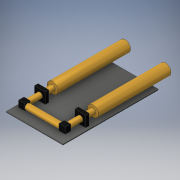
# Autodesk Inventor part: Cannon Barrel
Saved by Autodesk Inventor 2016 (Build 200138000, 138)
## iProperties
Created: 2018-05-17
Part Number: Cannon Barrel
Material: Generic
Document SubType Name: Modeling
Designer: Kade
Density: 1 g/cm^3
Appearance: Default
Mass: 6981.81 g
Surface Area: 8261.67 cm^2
Volume: 6981.81 cm^3
Author: Kade
Autodesk Inventor part; units mm, degrees
ref_plane "YZ Plane" through (0, 0, 0) normal (1, 0, 0) x (0, 1, 0)
ref_plane "XZ Plane" through (0, 0, 0) normal (0, 1, 0) x (-1, 0, 0)
ref_plane "XY Plane" through (0, 0, 0) normal (0, 0, 1) x (1, 0, 0)
sketch "Sketch1" plane through (0, 0, 0) normal (0, 1, 0) x (-1, 0, 0)
  line L0 (198.4375, 333.375) -> (198.4375, -333.375)
  line L1 (198.4375, -333.375) -> (-198.4375, -333.375)
  line L2 (-198.4375, -333.375) -> (-198.4375, 333.375)
  line L3 (-198.4375, 333.375) -> (198.4375, 333.375)
  line L4 (198.4375, 333.375) -> (-198.4375, -333.375) construction
  line L5 (198.4375, -333.375) -> (-198.4375, 333.375) construction
  point P0 (0, 0)
  dimension "d0" = 666.75
  dimension "d1" = 396.875
  constraints: 12 end point, 2 midpoint, 2 parallel, 1 perpendicular, 1 vertical
  measures "d0" distance of L0.start L0.end
  measures "d1" distance of L0.end L1.end
extrude "Extrusion1" add sketch "Sketch1" along normal blind 6.35
sketch "Sketch2" plane through (0, 6.35, 0) normal (0, 1, 0) x (1, 0, 0)
  line L0 (179.3875, -155.575) -> (103.1875, -155.575)
  line L1 (103.1875, -155.575) -> (103.1875, -130.175)
  line L2 (103.1875, -130.175) -> (179.3875, -130.175)
  line L3 (179.3875, -130.175) -> (179.3875, -155.575)
  line L4 (198.4375, -333.375) -> (198.4375, 333.375) projected
  line L5 (-179.3875, -155.575) -> (-103.1875, -155.575)
  line L6 (-103.1875, -155.575) -> (-103.1875, -130.175)
  line L7 (-103.1875, -130.175) -> (-179.3875, -130.175)
  line L8 (-179.3875, -130.175) -> (-179.3875, -155.575)
  line L9 (-198.4375, 333.375) -> (-198.4375, -333.375) projected
  line L10 (198.4375, -333.375) -> (-198.4375, -333.375) projected
  point P0 (0, 0)
  dimension "d4" = 76.2
  dimension "d5" = 25.4
  dimension "d6" = 19.05
  dimension "d7" = 76.2
  dimension "d8" = 25.4
  dimension "d9" = 19.05
  dimension "d10" = 177.8
  dimension "d11" = 177.8
  constraints: 16 end point, 4 parallel, 2 horizontal, 2 perpendicular
  measures "d4" distance of L1.end L2.end
  measures "d5" distance of L0.end L1.end
  measures "d6" distance between parallel lines of L3 L4
  measures "d7" distance of L7.end L6.end
  measures "d8" distance of L6.end L5.end
  measures "d9" distance between parallel lines of L9 L8
  measures "d10" distance between parallel lines of L10 L0
  measures "d11" distance between parallel lines of L10 L5
extrude "Extrusion2" add sketch "Sketch2" along normal blind 76.2
sketch "Sketch3" plane through (-179.3875, 6.35, 155.575) normal (0, 0, 1) x (1, 0, 0)
  circle A0 centre (38.1, 38.1) radius 19.05
  circle A1 centre (228.6, 38.1) radius 19.05
  point P0 (179.3875, -6.35)
  dimension "d14" = 38.1
  dimension "d15" = 38.1
  constraints: 2 centre point
  measures "d14" diameter of A0
  measures "d15" diameter of A1
extrude "Extrusion3" cut sketch "Sketch3" against normal blind 76.2
sketch "Sketch4" plane through (-179.3875, 6.35, 155.575) normal (0, 0, 1) x (1, 0, 0)
  circle A0 centre (38.1, 38.1) radius 19.05 projected
  circle A1 centre (38.1, 38.1) radius 19.05
  circle A2 centre (320.675, 38.1) radius 19.05
  point P0 (179.3875, -6.35)
  dimension "d44" = 38.1
  constraints: 2 centre point, 1 coincident
  measures "d44" diameter of A2
extrude "Extrusion4" add sketch "Sketch4" along normal blind 88.9 and the other way blind 88.9
sketch "Sketch5" plane through (49.2125, 44.45, 66.675) normal (0, 0, -1) x (-1, 0, 0)
  circle A0 centre (190.5, 0) radius 19.05 projected
  circle A1 centre (190.5, 0) radius 38.1
  circle A2 centre (-92.075, 0) radius 19.05 projected
  circle A3 centre (-92.075, 0) radius 38.1
  point P0 (49.2125, -44.45)
  dimension "d23" = 76.2
  constraints: 2 centre point, 2 coincident
  measures "d23" diameter of A1
extrude "Extrusion5" add sketch "Sketch5" along normal blind 508 contours A0 | A1 | A2 | A3
sketch "Sketch6" plane through (-141.2875, 44.45, 244.475) normal (0, 0, 1) x (1, 0, 0)
  line L0 (-22.225, -22.225) -> (22.225, -22.225)
  line L1 (22.225, -22.225) -> (22.225, 22.225)
  line L2 (22.225, 22.225) -> (-22.225, 22.225)
  line L3 (-22.225, 22.225) -> (-22.225, -22.225)
  line L4 (-22.225, -22.225) -> (22.225, 22.225) construction
  line L5 (22.225, -22.225) -> (-22.225, 22.225) construction
  line L6 (304.8, -22.225) -> (260.35, -22.225)
  line L7 (260.35, -22.225) -> (260.35, 22.225)
  line L8 (260.35, 22.225) -> (304.8, 22.225)
  line L9 (304.8, 22.225) -> (304.8, -22.225)
  line L10 (304.8, -22.225) -> (260.35, 22.225) construction
  line L11 (260.35, -22.225) -> (304.8, 22.225) construction
  line L12 (-38.1, -38.1) -> (-38.1, 38.1) projected
  line L13 (-38.1, 38.1) -> (38.1, 38.1) projected
  point P0 (141.2875, -44.45)
  point P1 (0, 0)
  point P2 (282.575, 0)
  dimension "d26" = 44.45
  dimension "d27" = 44.45
  dimension "d28" = 44.45
  dimension "d29" = 44.45
  dimension "d30" = 282.575
  dimension "d31" = 38.1
  dimension "d32" = 38.1
  constraints: 24 end point, 4 midpoint, 4 parallel, 2 horizontal, 2 perpendicular
  measures "d26" distance of L2.end L1.end
  measures "d27" distance of L1.end L0.end
  measures "d28" distance of L7.end L8.end
  measures "d29" distance of L6.end L7.end
  measures "d30" distance of point (282.575, 0) point (0, 0)
  measures "d31" distance from line of L12 point (0, 0)
  measures "d32" distance from line of L13 point (0, 0)
extrude "Extrusion6" add sketch "Sketch6" along normal blind 38.1
sketch "Sketch7" plane through (119.0625, 22.225, 244.475) normal (-1, 0, 0) x (0, 0, 1)
  circle A0 centre (19.05, 19.05) radius 19.05
  line L0 (0, 0) -> (0, 44.45) projected
  line L1 (0, 0) -> (38.1, 0) projected
  point P0 (-244.475, -22.225)
  dimension "d35" = 38.1
  dimension "d36" = 19.05
  dimension "d37" = 19.05
  constraints: 1 centre point
  measures "d35" diameter of A0
  measures "d36" distance from line of L0 A0.centre
  measures "d37" distance from line of L1 A0.centre
extrude "Extrusion7" add sketch "Sketch7" along normal blind 238.125 contours A0
sketch "Sketch9" plane through (-141.2875, 44.45, -441.325) normal (0, 0, -1) x (-1, 0, 0)
  circle A0 centre (0, 0) radius 36.5125
  point P0 (-141.2875, -44.45)
  dimension "d45" = 73.025
  constraints: 1 centre point
  measures "d45" diameter of A0
extrude "Extrusion9" cut sketch "Sketch9" against normal blind 501.65
body "Solid1"
